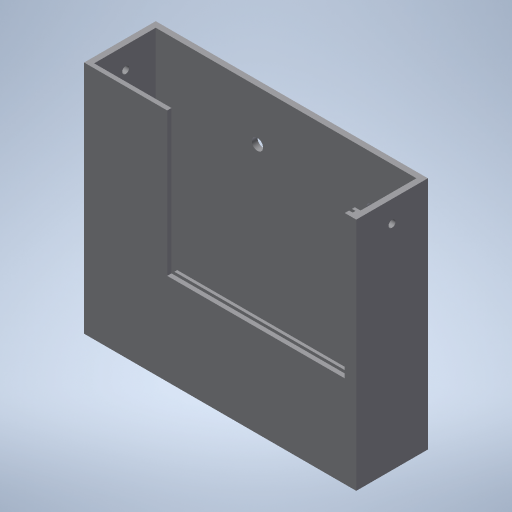
# Autodesk Inventor part: krab2
Saved by Autodesk Inventor 2023 (Build 270158000, 158)
## iProperties
Created: 2024-03-18
Part Number: krab2
Material: Všeobecné
Document SubType Name: Modeling
Designer: sok
Density: 1 g/cm^3
Appearance: Výchozí
Author: sok
Autodesk Inventor part; units mm, degrees
ref_plane "YZ Plane" through (0, 0, 0) normal (1, 0, 0) x (0, 1, 0)
ref_plane "XZ Plane" through (0, 0, 0) normal (0, 1, 0) x (-1, 0, 0)
ref_plane "XY Plane" through (0, 0, 0) normal (0, 0, 1) x (1, 0, 0)
sketch "Náčrt2" plane through (0, 0, 0) normal (0, 0, 1) x (1, 0, 0)
  line L0 (0, 0) -> (190, 0)
  line L1 (190, 0) -> (190, -50)
  line L2 (190, -50) -> (0, -50)
  line L3 (0, -50) -> (0, 0)
  dimension "d2" = 190
  dimension "d3" = 50
  constraints: 8 end point, 2 parallel, 1 horizontal, 1 perpendicular
  measures "d2" distance of L1.end L2.end
  measures "d3" distance of L0.end L1.end
extrude "Vysunutí2" add sketch "Náčrt2" along normal blind 4
sketch "Náčrt3" plane through (0, 0, 4) normal (0, 0, 1) x (1, 0, 0)
  line L0 (190, 0) -> (0, 0) projected
  line L1 (0, -50) -> (190, -50) projected
  line L2 (190, -50) -> (190, 0) projected
  line L3 (190, 0) -> (0, 0) projected
  line L4 (0, 0) -> (0, -50) projected
  line L5 (4, -46) -> (186, -46)
  line L6 (186, -46) -> (186, -4)
  line L7 (186, -4) -> (4, -4)
  line L8 (4, -4) -> (4, -46)
  dimension "d7" = 4
  constraints: 8 end point, 3 other
  measures "d7" distance between parallel lines of L4 L8
extrude "Vysunutí3" add sketch "Náčrt3" along normal blind 160
sketch "Náčrt4" plane through (0, -50, 0) normal (0, -1, 0) x (1, 0, 0)
  line L0 (4, 164) -> (186, 164) projected
  line L1 (182, 164) -> (58, 164)
  line L2 (58, 164) -> (58, 64)
  line L3 (58, 64) -> (182, 64)
  line L4 (182, 64) -> (182, 164)
  line L5 (190, 0) -> (190, 164) projected
  point P0 (0, 0)
  dimension "d10" = 8
  dimension "d11" = 100
  dimension "d12" = 124
  constraints: 8 end point, 2 parallel, 1 horizontal, 1 perpendicular, 1 point on line
  measures "d10" distance between parallel lines of L5 L4
  measures "d11" distance of L3.end L1.start
  measures "d12" distance of L2.end L3.end
extrude "Vysunutí4" cut sketch "Náčrt4" against normal blind 10
sketch "Náčrt5" plane through (4, -4, 4) normal (0, -1, 0) x (1, 0, 0)
  line L0 (54, 60) -> (54, 160) projected
  line L1 (178, 60) -> (54, 60) projected
  circle A0 centre (151, 125) radius 4
  circle A1 centre (71, 125) radius 4
  line L2 (186, -4) -> (186, 160) projected
  line L3 (0, 160) -> (182, 160) projected
  point P0 (-4, -4)
  dimension "d15" = 8
  dimension "d16" = 8
  dimension "d17" = 35
  dimension "d18" = 80
  dimension "d19" = 35
  dimension "d20" = 35
  constraints: 2 centre point
  measures "d15" diameter of A0
  measures "d16" diameter of A1
  measures "d17" distance from line of L2 A0.centre
  measures "d18" distance of A1.centre A0.centre
  measures "d19" distance from line of A0.centre L3
  measures "d20" distance from line of L3 A1.centre
extrude "Vysunutí5" cut sketch "Náčrt5" against normal blind 10
sketch "Náčrt6" plane through (4, -46, 4) normal (0, 1, 0) x (1, 0, 0)
  line L0 (-4, 4) -> (186, 4) projected
  line L1 (-4, 4) -> (-4, -160) projected
  line L2 (178, -160) -> (178, -60) projected
  line L3 (178, -60) -> (54, -60) projected
  line L4 (54, -60) -> (54, -160) projected
  line L5 (-4, -160) -> (54, -160) projected
  line L6 (-4, 4) -> (-4, -160) projected
  line L7 (-4, 4) -> (186, 4) projected
  line L8 (186, 4) -> (186, -160) projected
  line L9 (178, -160) -> (186, -160) projected
extrude "Vysunutí6" add sketch "Náčrt6" along normal blind 3
sketch "Náčrt7" plane through (0, 0, 164) normal (0, 0, 1) x (1, 0, 0)
  line L0 (184.5, -47) -> (4, -47)
  line L1 (4, -47) -> (4, -45)
  line L2 (4, -45) -> (184.5, -45)
  line L3 (184.5, -45) -> (184.5, -47)
  line L4 (182, -43) -> (182, -50) projected
  line L5 (182, -50) -> (190, -50) projected
  point P0 (0, 0)
  dimension "d25" = 2.5
  dimension "d26" = 2
  dimension "d27" = 3
  dimension "d28" = 180.5
  constraints: 8 end point, 2 parallel, 1 horizontal, 1 perpendicular
  measures "d25" distance between parallel lines of L3 L4
  measures "d26" distance of L2.end L0.start
  measures "d27" distance between parallel lines of L5 L0
  measures "d28" distance of L0.start L0.end
extrude "Vysunutí7" cut sketch "Náčrt7" against normal blind 105
sketch "Náčrt8" plane through (4, -43, 4) normal (0, 1, 0) x (1, 0, 0)
  line L0 (54, -160) -> (54, -60) projected
  line L1 (0, -160) -> (54, -160) projected
  line L2 (54, -160) -> (0, -160)
  line L3 (0, -160) -> (0, -60)
  line L4 (0, -60) -> (54, -60)
  line L5 (54, -60) -> (54, -160)
  point P0 (-4, 4)
  point P1 (54, -60)
  dimension "d31" = 54
  dimension "d32" = 100
  constraints: 8 end point, 2 parallel, 1 horizontal, 1 perpendicular
  measures "d31" distance of L3.end L4.end
  measures "d32" distance between parallel lines of L1 L4
extrude "Vysunutí8" cut sketch "Náčrt8" against normal up to surface (4 mm away)
sketch "Náčrt9" plane through (4, -43, 4) normal (0, 1, 0) x (1, 0, 0)
  line L0 (54, -60) -> (54, -160) projected
  line L1 (0, 0) -> (54, 0)
  line L2 (54, 0) -> (54, -60)
  line L3 (54, -60) -> (0, -60)
  line L4 (0, -60) -> (0, 0)
  point P0 (-4, 4)
  dimension "d35" = 54
  constraints: 8 end point, 2 parallel, 1 horizontal, 1 perpendicular
  measures "d35" distance of L1.start L1.end
extrude "Vysunutí9" cut sketch "Náčrt9" against normal blind 4
sketch "Náčrt10" plane through (190, -50, 0) normal (1, 0, 0) x (0, 0, -1)
  circle A0 centre (-149, 25) radius 2.5
  line L0 (0, 0) -> (-164, 0) projected
  line L1 (-164, 0) -> (-164, 50) projected
  point P0 (0, 50)
  dimension "d38" = 5
  dimension "d39" = 25
  dimension "d40" = 15
  constraints: 1 centre point
  measures "d38" diameter of A0
  measures "d39" distance from line of A0.centre L0
  measures "d40" distance from line of A0.centre L1
extrude "Vysunutí10" cut sketch "Náčrt10" against normal through all
sketch "Náčrt11" plane through (0, 0, 4) normal (0, 0, 1) x (1, 0, 0)
  circle A0 centre (25.2842, -14.6015) radius 2.5
  circle A1 centre (35.2842, -14.6015) radius 2.5
  circle A2 centre (45.2842, -14.6015) radius 2.5
  circle A3 centre (31.1056, -24.6015) radius 2.5
  circle A4 centre (41.1056, -24.6015) radius 2.5
  circle A5 centre (36.7049, -34.6015) radius 2.5
  line L0 (25.2842, -14.6015) -> (59.2692, -14.6015) construction
  line L1 (31.1056, -24.6015) -> (52.5835, -24.6015) construction
  point P0 (0, 0)
  dimension "d43" = 5
  dimension "d44" = 5
  dimension "d45" = 5
  dimension "d46" = 5
  dimension "d47" = 5
  dimension "d48" = 5
  dimension "d49" = 10
  dimension "d50" = 10
  dimension "d51" = 10
  dimension "d52" = 10
  dimension "d53" = 10
  constraints: 6 centre point, 4 end point, 3 point on line, 2 horizontal
  measures "d43" diameter of A0
  measures "d44" diameter of A1
  measures "d45" diameter of A2
  measures "d46" diameter of A3
  measures "d47" diameter of A4
  measures "d48" diameter of A5
  measures "d49" distance of A1.centre L0.start
  measures "d50" distance of A2.centre A1.centre
  measures "d51" distance of A4.centre L1.start
  measures "d52" distance between parallel lines of L1 L0
  measures "d53" distance from line of A5.centre L1
extrude "Vysunutí11" cut sketch "Náčrt11" against normal through all
pattern_linear "Obdélníkové pole1" count 3 spacing 55 along (1, 0, 0) of "Vysunutí11"
